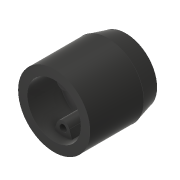
# Autodesk Inventor part: Cap no LED
Saved by Autodesk Inventor 2017 (Build 210142000, 142)
## iProperties
Created: 2016-08-05
Part Number: Cap no LED
Material: Generic
Document SubType Name: Modeling
Designer: ge937963
Density: 1 g/cm^3
Appearance: Smooth - Black
Mass: 7.97027 g
Surface Area: 42.9951 cm^2
Volume: 7.97027 cm^3
Author: ge937963
Autodesk Inventor part; units mm, degrees
ref_plane "YZ Plane" through (0, 0, 0) normal (1, 0, 0) x (0, 1, 0)
ref_plane "XZ Plane" through (0, 0, 0) normal (0, 1, 0) x (-1, 0, 0)
ref_plane "XY Plane" through (0, 0, 0) normal (0, 0, 1) x (1, 0, 0)
sketch "Sketch1" plane through (0, 0, 0) normal (0, 0, 1) x (1, 0, 0)
  circle A0 centre (0, 0) radius 12.7
  dimension "d0" = 25.4
  constraints: 1 centre point, 1 coincident
  measures "d0" diameter of A0
extrude "Extrusion1" add sketch "Sketch1" along normal blind 25.4
sketch "Sketch3" plane through (0, 0, 0) normal (0, 0, -1) x (-1, 0, 0)
  circle A0 centre (0, 0) radius 9.525
  dimension "d6" = 19.05
  constraints: 1 centre point, 1 coincident
  measures "d6" diameter of A0
extrude "Extrusion3" cut sketch "Sketch3" against normal blind 3.175
sketch "Sketch4" plane through (0, 0, 3.175) normal (0, 0, -1) x (-1, 0, 0)
  circle A0 centre (0, 0) radius 3.683
  circle A1 centre (0, 0) radius 9.525 projected
  arc A2 (-3.175, 8.9803) -> (3.175, 8.9803) centre (0, 0) ccw projected
  dimension "d40" = 7.366
  constraints: 1 centre point, 1 concentric
  measures "d40" diameter of A0
extrude "Extrusion4" cut sketch "Sketch4" against normal blind 5.2926 contours A0
sketch "Sketch5" plane through (0, 0, 25.4) normal (0, 0, 1) x (1, 0, 0)
  circle A0 centre (0, 0) radius 9.525
  dimension "d13" = 19.05
  constraints: 1 centre point, 1 coincident
  measures "d13" diameter of A0
extrude "Extrusion5" cut sketch "Sketch5" against normal blind 11.43
sketch "Sketch7" plane through (0, 0, 13.97) normal (0, 0, 1) x (1, 0, 0)
  circle A0 centre (0, 0) radius 3.683 projected
  circle A1 centre (-4.7625, 0) radius 3.429 projected
  circle A2 centre (-4.7625, 0) radius 1.6433
  circle A3 centre (0, 0) radius 4.572
  dimension "d47" = 9.144
  constraints: 2 centre point, 2 coincident
  measures "d47" diameter of A3
extrude "Extrusion8" cut sketch "Sketch7" against normal blind 3.81 contours A0 A1 | A0 A1 A3 | A1 A0 A2 | A0 A2 A3 A1 | A1 A3 A2 A0 | A2 A0 | A0 A2 A3
sketch "Sketch8" plane through (0, 0, 10.16) normal (0, 0, 1) x (1, 0, 0)
  circle A0 centre (0, 0) radius 2.754
  constraints: 1 centre point
extrude "Extrusion9" cut sketch "Sketch8" against normal through all
sketch "Sketch9" plane through (0, 0, 13.97) normal (0, 0, 1) x (1, 0, 0)
  circle A0 centre (0, -6.985) radius 2.286 projected
  circle A1 centre (0, 6.985) radius 2.286 projected
  circle A2 centre (0, 0) radius 9.525 projected
  line L0 (-2.1601, -6.2369) -> (-3.1173, -9.0005)
  line L1 (-2.1601, 6.2369) -> (-3.1173, 9.0005)
  line L2 (3.1173, -9.0005) -> (2.1601, -6.2369)
  line L3 (2.1601, 6.2369) -> (3.1173, 9.0005)
  constraints: 8 end point, 8 point on circle, 4 line through centre, 4 tangent
extrude "Extrusion10" add sketch "Sketch9" along normal blind 8.255 contours A0 | A0 L2 A2 L0 | A2 L3 A1 L1 | A1
sketch "Sketch10" plane through (0, 0, 22.225) normal (0, 0, 1) x (1, 0, 0)
  circle A0 centre (0, -6.985) radius 1.27
  circle A1 centre (0, 6.985) radius 1.27
  circle A2 centre (0, -6.985) radius 2.286 projected
  circle A3 centre (0, 6.985) radius 2.286 projected
  point P0 (0, 0)
  dimension "d28" = 2.54
  dimension "d29" = 2.54
  constraints: 2 centre point, 2 coincident
  measures "d28" diameter of A0
  measures "d29" diameter of A1
extrude "Extrusion11" cut sketch "Sketch10" against normal blind 7.62 contours A0 | A1
chamfer "Chamfer1" distance 6.35 angle 15 1 edges at (-12.7, 0, 0) measured on face at (12.6588, -1.0219, 16.9333)
sketch "Sketch12" plane through (0, 0, 3.175) normal (0, 0, -1) x (-1, 0, 0)
  circle A0 centre (5.9436, 0) radius 1.27
  circle A1 centre (-5.9436, 0) radius 1.27
  point P0 (0, 0)
  dimension "d41" = 2.54
  dimension "d42" = 2.54
  dimension "d43" = 5.9436
  dimension "d44" = 5.9436
  constraints: 2 centre point
  measures "d41" diameter of A0
  measures "d42" diameter of A1
  measures "d43" distance of A0.centre point (0, 0)
  measures "d44" distance of point (0, 0) A1.centre
extrude "Extrusion13" cut sketch "Sketch12" against normal blind 6.35
body "Solid1"
